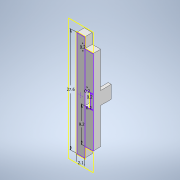
# Autodesk Inventor part: prototype7_2
Saved by Autodesk Inventor 2022 (Build 260153000, 153)
## iProperties
Created: 2022-06-15
Part Number: prototype7_2
Material: Generic
Document SubType Name: Modeling
Designer: tecware
Density: 1 g/cm^3
Appearance: Default
Author: tecware
Autodesk Inventor part; units mm, degrees
ref_plane "YZ Plane" through (0, 0, 0) normal (1, 0, 0) x (0, 1, 0)
ref_plane "XZ Plane" through (0, 0, 0) normal (0, 1, 0) x (-1, 0, 0)
ref_plane "XY Plane" through (0, 0, 0) normal (0, 0, 1) x (1, 0, 0)
sketch "Sketch1" plane through (0, 0, 0) normal (0, 0, 1) x (1, 0, 0)
  line L0 (0, 0) -> (0, -2.7) projected
  line L1 (0, -2.7) -> (-2.5, -2.7) projected
  line L2 (-2.5, -2.7) -> (-2.5, 25.3) projected
  line L3 (0, 25.3) -> (-2.5, 25.3) projected
  line L4 (0, 25.3) -> (0, 22.6) projected
  line L5 (0, 22.6) -> (2, 22.6) projected
  line L6 (2, 27.3) -> (2, 22.6) projected
  line L7 (-4.5, 27.3) -> (2, 27.3) projected
  line L8 (-4.5, -4.7) -> (-4.5, 27.3) projected
  line L9 (-4.5, -4.7) -> (2, -4.7) projected
  line L10 (2, 0) -> (2, -4.7) projected
  line L11 (0, 0) -> (2, 0) projected
  line L12 (-0.2, 25.1) -> (-2.3, 25.1)
  line L13 (-2.3, 25.1) -> (-2.3, -2.5)
  line L14 (-2.3, -2.5) -> (-0.2, -2.5)
  line L15 (-0.2, -2.5) -> (-0.2, 25.1)
  line L16 (0, 22.6) -> (0, 22.4) construction
  line L17 (1, 13) -> (2, 13) projected
  line L18 (1, 9.6) -> (1, 13) projected
  line L19 (2, 9.6) -> (1, 9.6) projected
  line L20 (2, 13) -> (2, 9.6) projected
  line L21 (1, 11.3) -> (1.2, 11.3) construction
  line L22 (2, 13) -> (1.2, 13)
  line L23 (1.2, 13) -> (1.2, 9.6)
  line L24 (1.2, 9.6) -> (2, 9.6)
  line L25 (2, 9.6) -> (2, 13)
  line L26 (1.2, 13) -> (1.2, 13.2)
  line L27 (2, 13.2) -> (-0.2, 13.2)
  line L28 (-0.2, 13.2) -> (-0.2, 22.4)
  line L29 (-0.2, 22.4) -> (2, 22.4)
  line L30 (2, 22.4) -> (2, 13.2)
  line L31 (2, 13.2) -> (2, 13)
  line L32 (2, 9.6) -> (1.2, 9.6)
  line L33 (1.2, 9.6) -> (1.2, 9.4)
  line L34 (1.2, 9.4) -> (2, 9.4)
  line L35 (2, 9.4) -> (2, 9.6)
  line L36 (2, 9.4) -> (-0.2, 9.4)
  line L37 (-0.2, 9.4) -> (-0.2, 0.2)
  line L38 (-0.2, 0.2) -> (2, 0.2)
  line L39 (2, 0.2) -> (2, 9.4)
  point P0 (-1.25, 11.3)
  point P1 (-1.25, 11.3)
  dimension "d0" = 2.1
  dimension "d1" = 27.6
  dimension "d2" = 0.2
  dimension "d3" = 0.2
  dimension "d4" = 0.2
  dimension "d5" = 0.2
  dimension "d6" = 9.2
  constraints: 48 end point, 3 point on line, 1 midpoint
  measures "d0" distance of L14.end L13.end
  measures "d1" distance of L13.end L12.end
  measures "d2" distance of L4.end L16.end
  measures "d3" distance of L21.start L21.end
  measures "d4" distance of L22.end L26.end
  measures "d5" distance of L33.end L32.end
  measures "d6" distance of L37.end L36.end
extrude "Extrusion1" add sketch "Sketch1" against normal blind 2 contours L15 L14 L13 L12 | L29 L30 L27 L15 | L36 L34 L39 L38 L15 | L27 L31 L17 L26 | L33 L19 L35 L34 | L17 L20 L19 L23
sketch "Sketch2" plane through (2, 0.2, 0) normal (1, 0, 0) x (0, 0, -1)
  arc A0 (9, -0.2) -> (9, 9.4) centre (9, 4.6) ccw projected
  arc A1 (9, 12.8) -> (9, 22.4) centre (9, 17.6) ccw projected
  circle A2 centre (9, 4.6) radius 4.6
  circle A3 centre (9, 17.6) radius 4.6
  line L0 (2, 22.2) -> (2, 0) projected
  line L1 (9, 0) -> (2, 0)
  line L2 (9, 9.2) -> (2, 9.2)
  line L3 (2, 0) -> (2, 9.2)
  line L4 (9, 13) -> (2, 13)
  line L5 (2, 13) -> (2, 22.2)
  line L6 (0, 22.2) -> (2, 22.2) projected
  line L7 (9, 22.2) -> (2, 22.2)
  point P0 (0, -0.2)
  dimension "d12" = 9.2
  dimension "d13" = 9.2
  constraints: 12 end point, 4 point on circle, 2 centre point, 2 coincident, 1 point on line
  measures "d12" diameter of A2
  measures "d13" diameter of A3
extrude "Extrusion3" add sketch "Sketch2" against normal blind 2 contours A2 L1 L0 L2 | A3 L4 L0 L7
body "Solid1"
